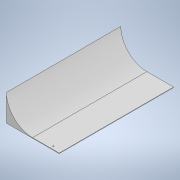
# Autodesk Inventor part: 零件2
Saved by Autodesk Inventor 2020 (Build 240168000, 168)
## iProperties
Created: 2020-12-03
Part Number: 零件2
Material: 常规
Document SubType Name: Sheet Metal
Designer: huang
Density: 1 g/cm^3
Sheet Metal Rule: 默认_mm
Appearance: 默认
Author: huang
Autodesk Inventor part; units mm, degrees
ref_plane "YZ Plane" through (0, 0, 0) normal (1, 0, 0) x (0, 1, 0)
ref_plane "XZ Plane" through (0, 0, 0) normal (0, 1, 0) x (-1, 0, 0)
ref_plane "XY Plane" through (0, 0, 0) normal (0, 0, 1) x (1, 0, 0)
sketch "草图1" plane through (0, 0, 0) normal (0, 1, 0) x (-1, 0, 0)
  line L0 (44.8045, 618.8377) -> (-43.3955, 618.8377)
  line L1 (-43.3955, 618.8377) -> (-43.3955, -101.1623)
  line L2 (-43.3955, -101.1623) -> (44.8045, -101.1623)
  line L3 (44.8045, -101.1623) -> (44.8045, 618.8377)
  point P0 (0, 0)
  dimension "d0" = 88.2
  dimension "d1" = 720
  constraints: 8 end point, 2 parallel, 1 horizontal, 1 perpendicular
  measures "d0" distance of L1.end L2.end
  measures "d1" distance of L2.end L0.start
extrude "拉伸1" add sketch "草图1" along normal blind 90
sketch "草图3" plane through (-44.8045, 0, 618.8377) normal (0, 0, 1) x (1, 0, 0)
  line L0 (88.2, 0) -> (88.2, 90) projected
  circle A0 centre (88.2, 90) radius 88.2
  line L1 (0, 0) -> (0, 90) projected
  point P0 (44.8045, 0)
  constraints: 1 horizontal alignment, 1 vertical, 1 other
extrude "拉伸3" cut sketch "草图3" against normal through all
sketch "草图4" plane through (-44.8045, 0, -101.1623) normal (-1, 0, 0) x (0, 0, 1)
  line L0 (0, 0) -> (0, 90) projected
  line L1 (0, 90) -> (5, 90)
  line L2 (0, 90) -> (720, 90) projected
  line L3 (5, 90) -> (75, 90)
  line L4 (75, 90) -> (75, 20)
  line L5 (5, 90) -> (5, 20)
  line L6 (5, 20) -> (75, 20)
  point P0 (101.1623, 0)
  dimension "d8" = 5
  dimension "d9" = 70
  dimension "d10" = 70
  constraints: 10 end point, 2 perpendicular, 2 point on line, 1 vertical
  measures "d8" distance of L0.end L1.end
  measures "d9" distance of L1.end L3.end
  measures "d10" distance of L3.end L4.end
extrude "拉伸4" cut sketch "草图4" against normal blind 90
sketch "草图5" plane through (43.3955, 0, -101.1623) normal (0, 0, -1) x (-1, 0, 0)
  line L0 (0, 0) -> (88.2, 0) projected
  line L1 (0, 0) -> (88.2, 0)
  line L2 (88.2, 0) -> (88.2, 90) projected
  line L3 (88.2, 0) -> (88.2, 90)
  arc A0 (0, 1.8) -> (88.2, 90) centre (0, 90) ccw projected
  arc A1 (0, 1.8) -> (88.2, 90) centre (0, 90) ccw
  line L4 (0, 0) -> (0, 1.8) projected
  line L5 (0, 1.8) -> (0, 0)
  point P0 (43.3955, 0)
  constraints: 6 end point, 3 point on circle, 2 collinear, 1 centre point, 1 horizontal, 1 point on line, 1 tangent
extrude "拉伸5" cut sketch "草图5" against normal blind 334
sketch "草图6" plane through (43.3955, 0, 618.8377) normal (1, 0, 0) x (0, 0, -1)
  line L0 (386, 1.8) -> (0, 1.8) projected
  line L1 (386, 0) -> (386, 1.8) projected
  line L2 (0, 1.8) -> (386, 1.8)
  line L3 (386, 1.8) -> (386, 0)
  line L4 (386, 0) -> (0, 0)
  line L5 (0, 0) -> (0, 1.8)
  point P0 (618.8377, 0)
  constraints: 8 end point, 2 parallel, 1 horizontal, 1 perpendicular
extrude "拉伸6" add sketch "草图6" along normal blind 90
sketch "草图7" plane through (43.3955, 1.8, 618.8377) normal (0, 1, 0) x (1, 0, 0)
  line L0 (-88.2, 0) -> (90, 0) projected
  line L1 (90, 0) -> (90, 10)
  line L2 (90, 0) -> (90, 386) projected
  line L3 (90, 10) -> (60, 10)
  circle A0 centre (60, 10) radius 2
  point P0 (-43.3955, 618.8377)
  dimension "d17" = 10
  dimension "d18" = 30
  dimension "d19" = 4
  constraints: 4 end point, 1 centre point, 1 coincident, 1 horizontal, 1 point on line
  measures "d17" distance of L0.end L1.end
  measures "d18" distance of L1.end L3.end
  measures "d19" diameter of A0
extrude "拉伸7" cut sketch "草图7" against normal blind 90
equation "\"折弯半径\" = 厚度"
equation "\"折弯释压宽度\" = 厚度"
equation "\"折弯释压深度\" = 0.5 * 厚度"
equation "\"拐角释压尺寸\" = 4 * 厚度"
equation "\"最小余量\" = 2 * 厚度"
equation "\"过渡半径\" = 折弯半径"
equation "\"Jacobi半径尺寸\" = 折弯半径"
equation "\"间隙大小\" = 厚度"
equation "\"厚度\" = 0.5"
